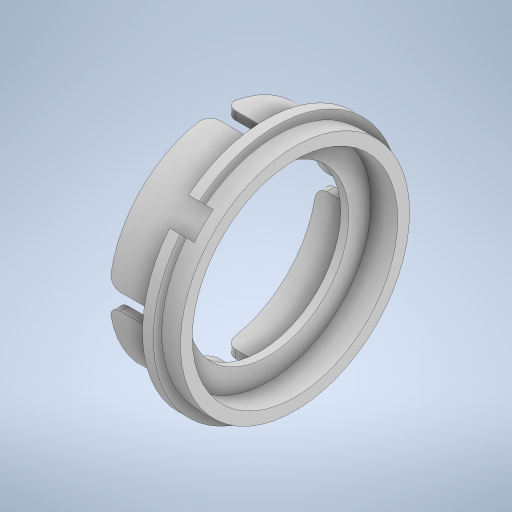
# Autodesk Inventor part: Parte3
Saved by Autodesk Inventor 2024 (Build 280153000, 153)
## iProperties
Created: 2023-12-18
Part Number: Parte3
Material: Generico
Document SubType Name: Modeling
Designer: cecca
Density: 1 g/cm^3
Appearance: Default
Author: cecca
Autodesk Inventor part; units mm, degrees
ref_plane "YZ Plane" through (0, 0, 0) normal (1, 0, 0) x (0, 1, 0)
ref_plane "XZ Plane" through (0, 0, 0) normal (0, 1, 0) x (-1, 0, 0)
ref_plane "XY Plane" through (0, 0, 0) normal (0, 0, 1) x (1, 0, 0)
sketch "Schizzo1" plane through (0, 0, 0) normal (1, 0, 0) x (0, 1, 0)
  circle A0 centre (0, 0) radius 18.5
  circle A1 centre (0, 0) radius 20
  dimension "d0" = 37
  dimension "d1" = 40
  constraints: 2 centre point, 2 coincident
  measures "d0" diameter of A0
  measures "d1" diameter of A1
sketch "Schizzo1 outline for Estrusione1" plane through (0, 0, 0) normal (1, 0, 0) x (0, 1, 0)
  circle A0 centre (0, 0) radius 20
  circle A1 centre (0, 0) radius 18.5
extrude "Estrusione1" add sketch "Schizzo1 outline for Estrusione1" along normal mid plane 9
sketch "Schizzo2" plane through (4.5, 0, 0) normal (1, 0, 0) x (0, 0, -1)
  circle A0 centre (0, 0) radius 22.85
  circle A1 centre (0, 0) radius 18.5
  dimension "d4" = 45.7
  constraints: 2 centre point, 2 coincident
  measures "d4" diameter of A0
sketch "Schizzo2 outline for Estrusione2" plane through (4.5, 0, 0) normal (1, 0, 0) x (0, 0, -1)
  circle A0 centre (0, 0) radius 22.85
  circle A1 centre (0, 0) radius 18.5
extrude "Estrusione2" add sketch "Schizzo2 outline for Estrusione2" along normal blind 2
sketch "Schizzo3" plane through (6.5, 0, 0) normal (1, 0, 0) x (0, 0, -1)
  circle A0 centre (0, 0) radius 19.1
  circle A1 centre (0, 0) radius 21.3
  dimension "d7" = 38.2
  dimension "d8" = 42.6
  constraints: 2 centre point, 2 coincident
  measures "d7" diameter of A0
  measures "d8" diameter of A1
sketch "Schizzo3 outline for Estrusione3" plane through (6.5, 0, 0) normal (1, 0, 0) x (0, 0, -1)
  circle A0 centre (0, 0) radius 21.3
  circle A1 centre (0, 0) radius 19.1
extrude "Estrusione3" add sketch "Schizzo3 outline for Estrusione3" along normal blind 3.5
sketch "Schizzo4" plane through (-4.5, 0, 0) normal (-1, 0, 0) x (0, 0, 1)
  line L0 (1.5, -25) -> (-1.5, -25)
  line L1 (-1.5, -25) -> (-1.5, 25)
  line L2 (-1.5, 25) -> (1.5, 25)
  line L3 (1.5, 25) -> (1.5, -25)
  line L4 (1.5, -25) -> (-1.5, 25) construction
  line L5 (-1.5, -25) -> (1.5, 25) construction
  point P0 (0, 0)
  dimension "d11" = 3
  dimension "d12" = 50
  constraints: 12 end point, 2 midpoint, 2 parallel, 1 horizontal, 1 perpendicular
  measures "d11" distance of L1.end L2.end
  measures "d12" distance of L0.end L1.end
sketch "Schizzo4 outline for Estrusione4" plane through (-4.5, 0, 0) normal (-1, 0, 0) x (0, 0, 1)
  line L0 (1.5, -25) -> (1.5, 25)
  line L1 (-1.5, -25) -> (1.5, -25)
  line L2 (-1.5, 25) -> (-1.5, -25)
  line L3 (1.5, 25) -> (-1.5, 25)
extrude "Estrusione4" cut sketch "Schizzo4 outline for Estrusione4" against normal blind 8
pattern_circular "Serie circolare1" count 2 over 90 about axis through (0, 0, 0) along (1, 0, 0) of "Estrusione4"
sketch "Schizzo5" plane through (3.5, 0, 0) normal (-1, 0, 0) x (0, 0, 1)
  circle A0 centre (0, 0) radius 15
  circle A1 centre (0, 0) radius 19.25
  dimension "d18" = 30
  dimension "d19" = 38.5
  constraints: 2 centre point, 2 coincident
  measures "d18" diameter of A0
  measures "d19" diameter of A1
sketch "Schizzo5 outline for Estrusione5" plane through (3.5, 0, 0) normal (-1, 0, 0) x (0, 0, 1)
  circle A0 centre (0, 0) radius 19.25
  circle A1 centre (0, 0) radius 15
extrude "Estrusione5" add sketch "Schizzo5 outline for Estrusione5" against normal blind 3
sketch "Schizzo6" plane through (10, 0, 0) normal (1, 0, 0) x (0, 0, -1)
  circle A0 centre (0, 0) radius 19.1
  constraints: 1 centre point, 1 coincident
sketch "Schizzo6 outline for Estrusione6" plane through (10, 0, 0) normal (1, 0, 0) x (0, 0, -1)
  circle A0 centre (0, 0) radius 19.1
extrude "Estrusione6" cut sketch "Schizzo6 outline for Estrusione6" against normal blind 5
sketch "Schizzo8" plane through (-4.5, 0, 0) normal (-1, 0, 0) x (0, 0, 1)
  line L0 (0, 0) -> (-21.213203, -21.213203)
  line L1 (0, 0) -> (30, 0) construction
  line L2 (-21.213203, -21.213203) -> (-22.98097, -19.445436)
  line L3 (-22.98097, -19.445436) -> (19.445436, 22.98097)
  line L4 (19.445436, 22.98097) -> (22.98097, 19.445436)
  line L5 (22.98097, 19.445436) -> (-19.445436, -22.98097)
  line L6 (-19.445436, -22.98097) -> (-21.213203, -21.213203)
  circle A0 centre (0, 0) radius 20
  circle A1 centre (0, 0) radius 23.148527
  point P0 (-14.504976, -18.04051)
  point P1 (-12.263448, -15.798982)
  point P2 (-15.798982, -12.263448)
  point P3 (-18.04051, -14.504976)
  point P4 (18.04051, 14.504976)
  point P5 (14.504976, 18.04051)
  point P6 (12.263448, 15.798982)
  point P7 (15.798982, 12.263448)
  dimension "d31" = 30
  dimension "d32" = 135
  dimension "d33" = 2.5
  dimension "d34" = 60
  dimension "d35" = 90
  dimension "d37" = 5
  constraints: 14 end point, 4 perpendicular, 2 centre point, 1 coincident, 1 equal length, 1 horizontal, 1 point on line
  measures "d31" distance of L0.start L0.end
  measures "d32" angle of L0 L1
  measures "d33" distance of L0.end L2.end
  measures "d34" distance of L2.end L3.end
  measures "d35" angle of L2 L3
  measures "d37" distance of L3.end L4.end
sketch "Schizzo8 outline for Estrusione7" plane through (-4.5, 0, 0) normal (-1, 0, 0) x (0, 0, 1)
  arc A0 (-18.04051, -14.504976) -> (-14.504976, -18.04051) centre (0, 0) ccw
  line L0 (-15.798982, -12.263448) -> (-18.04051, -14.504976)
  arc A1 (-12.263448, -15.798982) -> (-15.798982, -12.263448) centre (0, 0) cw
  line L1 (-14.504976, -18.04051) -> (-12.263448, -15.798982)
  arc A2 (18.04051, 14.504976) -> (14.504976, 18.04051) centre (0, 0) ccw
  line L2 (15.798982, 12.263448) -> (18.04051, 14.504976)
  arc A3 (12.263448, 15.798982) -> (15.798982, 12.263448) centre (0, 0) cw
  line L3 (14.504976, 18.04051) -> (12.263448, 15.798982)
extrude "Estrusione7" cut sketch "Schizzo8 outline for Estrusione7" against normal blind 12.5
fillet "Raccordo1" radius 2 8 edges at (-4.5, 1.5, -19.1914) (-4.5, 1.5, 19.1914) (-4.5, -1.5, -19.1914) (-4.5, -1.5, 19.1914) (-4.5, -19.1914, -1.5) (-4.5, 19.1914, -1.5) (-4.5, -19.1914, 1.5) (-4.5, 19.1914, 1.5)
